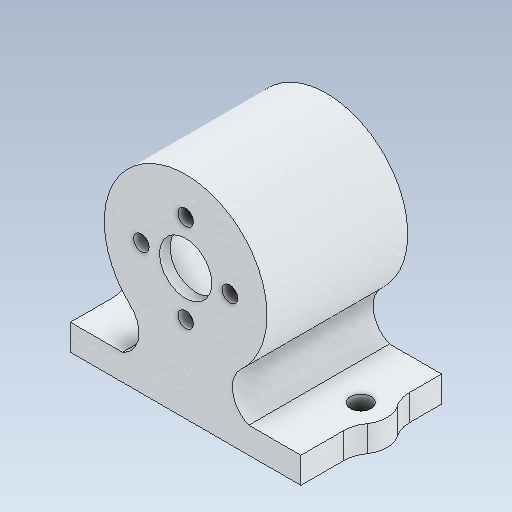
# Autodesk Inventor part: BaseM1
Saved by Autodesk Inventor 2021 (Build 250183000, 183)
## iProperties
Created: 2022-10-28
Part Number: BaseM1
Material: Generic
Document SubType Name: Modeling
Designer: zulet
Density: 1 g/cm^3
Appearance: White
Mass: 16.767 g
Surface Area: 88.0452 cm^2
Volume: 16.767 cm^3
Author: zulet
Autodesk Inventor part; units mm, degrees
ref_plane "YZ Plane" through (0, 0, 0) normal (1, 0, 0) x (0, 1, 0)
ref_plane "XZ Plane" through (0, 0, 0) normal (0, 1, 0) x (-1, 0, 0)
ref_plane "XY Plane" through (0, 0, 0) normal (0, 0, 1) x (1, 0, 0)
sketch "Sketch1" plane through (0, 0, 0) normal (0, 0, 1) x (1, 0, 0)
  circle A0 centre (0, 0) radius 12.12 projected
  circle A1 centre (0, 0) radius 12.62
  arc A2 (10.6143, -11.4595) -> (-10.6143, -11.4595) centre (0, 0) ccw
  line L0 (-12.12, -25) -> (12.12, -25)
  line L1 (12.12, 0) -> (12.12, -25.5944) construction
  line L2 (-12.12, 0) -> (-12.12, -25) construction
  line L3 (-12.12, -25) -> (12.12, -25)
  line L4 (12.12, -25) -> (12.12, -20)
  line L5 (12.12, -20) -> (-12.12, -20)
  line L6 (-12.12, -20) -> (-12.12, -25)
  arc A3 (-12.12, -20) -> (-10.6143, -11.4595) centre (-14.12, -15.2444) ccw
  line L7 (0, 0) -> (0, 15.62) construction
  arc A4 (10.6143, -11.4595) -> (12.12, -20) centre (14.12, -15.2444) ccw
  point P0 (12.12, -25)
  dimension "d0" = 0.5
  dimension "d1" = 3
  dimension "d2" = 25
  dimension "d3" = 5
  dimension "d4" = 2
  constraints: 16 end point, 9 point on circle, 4 centre point, 3 tangent, 3 vertical, 2 horizontal, 2 parallel, 2 perpendicular, 2 point on line, 2 symmetric about line, 1 other
  measures "d0" radial gap between concentric circles of A0 A1
  measures "d1" radial gap between concentric circles of A1 A2
  measures "d2" distance from line of L0 point (0, 0)
  measures "d3" distance of L4.end L3.end
  measures "d4" distance from line of L2 A3.centre
extrude "Extrusion1" add sketch "Sketch1" against normal blind 25 contours A4 L5 A3 A2 | L4 L0 L6 L5
sketch "Sketch2" plane through (12.12, -25, 0) normal (1, 0, 0) x (0, 0, -1)
  line L0 (0, 0) -> (0, 5) projected
  line L1 (0, 0) -> (25, 0) projected
  line L2 (25, 5) -> (25, 0) projected
  line L3 (0, 5) -> (25, 5) projected
  point P0 (0, 25)
extrude "Extrusion2" add sketch "Sketch2" along normal blind 10
sketch "Sketch3" plane through (-12.12, -25, 0) normal (-1, 0, 0) x (0, 0, 1)
  line L0 (0, 5) -> (0, 0) projected
  line L1 (0, 5) -> (-25, 5) projected
  line L2 (-25, 0) -> (-25, 5) projected
  line L3 (0, 0) -> (-25, 0) projected
  point P0 (0, 25)
extrude "Extrusion3" add sketch "Sketch3" along normal blind 10
sketch "Sketch4" plane through (12.12, -20, 0) normal (0, 1, 0) x (1, 0, 0)
  circle A0 centre (7, 12.5) radius 2
  circle A1 centre (-31.24, 12.5) radius 2
  line L0 (7, 12.5) -> (-31.24, 12.5) construction
  line L1 (10, 25) -> (10, 0) projected
  line L2 (7, 12.5) -> (10, 12.5) construction
  line L3 (10, 0) -> (10, 25) projected
  line L4 (-34.24, 0) -> (-34.24, 25) projected
  circle A2 centre (7, 12.5) radius 5
  circle A3 centre (-31.24, 12.5) radius 5
  point P0 (-12.12, 0)
  point P1 (-34.24, 16.5)
  point P2 (-34.24, 8.5)
  point P3 (10, 16.5)
  point P4 (10, 8.5)
  dimension "d11" = 4
  dimension "d12" = 4
  dimension "d13" = 3
  dimension "d14" = 3
  dimension "d17" = 10
  dimension "d18" = 10
  constraints: 4 centre point, 4 end point, 2 coincident, 2 horizontal, 1 midpoint
  measures "d11" diameter of A0
  measures "d12" diameter of A1
  measures "d13" distance from line of L1 L0.start
  measures "d14" distance from line of L4 L0.end
  measures "d17" diameter of A2
  measures "d18" diameter of A3
extrude "Extrusion4" cut sketch "Sketch4" against normal through all contours A0 | A1
extrude "Extrusion5" add sketch "Sketch4" against normal up to surface (5 mm away) contours A2 L1 | A3 L4 picked at (10.2796, 11.4321) picked at (-35.0103, 13.5108)
fillet "Fillet1" radius 6 4 edges at (22.12, -22.5, -8.5) (22.12, -22.5, -16.5) (-22.12, -22.5, -8.5) (-22.12, -22.5, -16.5)
sketch "Sketch5" plane through (0, 0, 0) normal (0, 0, 1) x (1, 0, 0)
  arc A0 (10.6143, -11.4595) -> (-10.6143, -11.4595) centre (0, 0) ccw projected
  arc A1 (-12.12, -20) -> (-10.6143, -11.4595) centre (-14.12, -15.2444) ccw projected
  line L0 (-12.12, -20) -> (-22.12, -20) projected
  line L1 (-22.12, -25) -> (-22.12, -20) projected
  line L2 (-22.12, -25) -> (22.12, -25) projected
  line L3 (22.12, -20) -> (22.12, -25) projected
  line L4 (12.12, -20) -> (22.12, -20) projected
  arc A2 (10.6143, -11.4595) -> (12.12, -20) centre (14.12, -15.2444) ccw projected
  circle A3 centre (0, 0) radius 12.62 projected
  circle A4 centre (0, 0) radius 8.5 construction
  circle A5 centre (0, 8.5) radius 1.5
  line L5 (0, 0) -> (0, 8.5) construction
  circle A6 centre (-8.5, 0) radius 1.5
  circle A7 centre (0, -8.5) radius 1.5
  circle A8 centre (8.5, 0) radius 1.5
  circle A9 centre (0, 0) radius 5
  dimension "d22" = 17
  dimension "d23" = 3
  dimension "d26" = 360
  dimension "d28" = 10
  constraints: 5 centre point, 2 coincident, 2 end point, 1 vertical, 1 vertical alignment, 11 other
  measures "d23" diameter of A5
  measures "d28" diameter of A9
extrude "Extrusion6" add sketch "Sketch5" along normal blind 2 contours A2 L4 L3 L2 L1 L0 A1 A0 | A3
equation "\"d1\" = TB"
equation "\"d2\" = HSE"
equation "\"d5\" = PB"
equation "\"DER\" = 22"
equation "\"HR\" = 7"
equation "\"DIR\" = 8"
equation "\"DEM\" = 4"
equation "\"Dmarc\" = 17.5"
equation "\"Bsm\" = 22.5"
equation "\"Hsm\" = 12"
equation "\"Lsm\" = 21"
equation "\"Dsc\" = 5"
equation "\"RC\" = 7"
equation "\"TB\" = 3"
equation "\"HSE\" = 25"
equation "\"PB\" = 25"
equation "\"LMaSP\" = 46.5"
body "Solid1"
